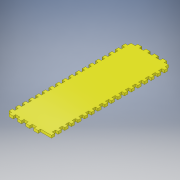
# Autodesk Inventor part: 000.203 - Боковая стенка лицевая
Saved by Autodesk Inventor 2019 (Build 230136000, 136)
## iProperties
Created: 2020-02-27
Part Number: 000.203 - Боковая стенка лицевая
Material: Типовые
Document SubType Name: Modeling
Designer: Петров Иван
Density: 1 g/cm^3
Appearance: Желтый
Author: Петров Иван
Autodesk Inventor part; units mm, degrees
ref_plane "YZ Plane" through (0, 0, 0) normal (1, 0, 0) x (0, 1, 0)
ref_plane "XZ Plane" through (0, 0, 0) normal (0, 1, 0) x (-1, 0, 0)
ref_plane "XY Plane" through (0, 0, 0) normal (0, 0, 1) x (1, 0, 0)
sketch "Эскиз1" plane through (0, 0, 0) normal (0, 1, 0) x (-1, 0, 0)
  line L0 (-22.5, 72) -> (22.5, 72)
  line L1 (22.5, 72) -> (22.5, -72)
  line L2 (22.5, -72) -> (-22.5, -72)
  line L3 (-22.5, -72) -> (-22.5, 72)
  line L4 (-22.5, 72) -> (22.5, -72) construction
  line L5 (22.5, 72) -> (-22.5, -72) construction
  point P0 (0, 0)
  point P1 (0, 0)
  dimension "d0" = 45
  dimension "d1" = 144
  constraints: 12 end point, 3 midpoint, 2 parallel, 1 horizontal, 1 perpendicular, 1 other
  measures "d0" distance of L1.end L2.end
  measures "d1" distance of L0.end L1.end
extrude "Выдавливание1" add sketch "Эскиз1" along normal blind 3
sketch "Эскиз2" plane through (0, 3, 0) normal (0, 1, 0) x (0, 0, -1)
  line L0 (-72, -22.5) -> (72, -22.5) projected
  line L1 (-72, -22.5) -> (-68, -22.5)
  line L2 (-68, -22.5) -> (-68, -25.5)
  line L3 (-68, -25.5) -> (-72, -25.5)
  line L4 (-72, -25.5) -> (-72, -22.5)
  point P0 (0, 0)
  dimension "d5" = 4
  dimension "d6" = 3
  constraints: 8 end point, 2 parallel, 1 horizontal, 1 perpendicular
  measures "d5" distance of L2.end L3.end
  measures "d6" distance of L1.end L2.end
extrude "Выдавливание2" add sketch "Эскиз2" against normal blind 3
pattern_linear "Прямоуг.массив1" count 18 spacing 8 along (0, 0, -1) of "Выдавливание2"
sketch "Эскиз3" plane through (0, 3, 0) normal (0, 1, 0) x (0, 0, -1)
  line L0 (72, 22.5) -> (-72, 22.5) projected
  line L1 (-72, 22.5) -> (-75, 22.5)
  line L2 (-75, 22.5) -> (-75, 17.5)
  line L3 (-75, 17.5) -> (-72, 17.5)
  line L4 (-72, 17.5) -> (-72, 22.5)
  line L5 (72, -22.5) -> (72, 22.5) projected
  line L6 (72, 17.5) -> (75, 17.5)
  line L7 (75, 17.5) -> (75, 12.5)
  line L8 (75, 12.5) -> (72, 12.5)
  line L9 (72, 12.5) -> (72, 17.5)
  point P0 (0, 0)
  dimension "d17" = 3
  dimension "d18" = 5
  dimension "d15" = 3
  dimension "d16" = 5
  dimension "d14" = 5
  constraints: 16 end point, 4 parallel, 2 horizontal, 2 perpendicular, 1 point on line
  measures "d17" distance of L3.end L2.end
  measures "d18" distance of L2.end L1.end
  measures "d15" distance of L7.end L8.end
  measures "d16" distance of L6.end L7.end
  measures "d14" distance between parallel lines of L0 L6
extrude "Выдавливание3" add sketch "Эскиз3" against normal blind 3
pattern_linear "Прямоуг.массив2" count 4 spacing 10 along (1, 0, 0) of "Выдавливание3"
sketch "Эскиз4" plane through (0, 3, 0) normal (0, 1, 0) x (1, 0, 0)
  line L0 (-9.4334, -33.577) -> (-9.4334, 33.2438) construction
  line L1 (-9.4334, 33.2438) -> (8.0885, 33.2438) construction
  line L2 (8.0885, 33.2438) -> (8.0885, -33.577) construction
  line L3 (8.0885, -33.577) -> (-9.4334, -33.577) construction
  point P0 (0, 0)
  constraints: 2 other
sketch "Эскиз5" plane through (0, 0, 0) normal (0, -1, 0) x (1, 0, 0)
  line L0 (-9.4334, -33.577) -> (-9.4334, 33.2438) construction
  line L1 (-9.4334, 33.2438) -> (8.0885, 33.2438) construction
  line L2 (8.0885, 33.2438) -> (8.0885, -33.577) construction
  line L3 (8.0885, -33.577) -> (-9.4334, -33.577) construction
  line L4 (8.0885, -18.72) -> (8.0885, -28.0611)
  line L5 (8.0885, -28.0611) -> (5.0082, -31.256)
  line L6 (5.0082, -31.256) -> (-6.3244, -31.256)
  line L7 (-6.3244, -31.256) -> (-9.4334, -28.0611)
  line L8 (-9.4334, -28.0611) -> (-9.4334, -18.9206)
  line L9 (-9.4334, -18.9206) -> (-8.0723, -18.9206)
  line L10 (-8.0723, -18.9206) -> (-8.0723, -27.5024)
  line L11 (-8.0723, -27.5024) -> (-5.7943, -29.852)
  line L12 (-5.7943, -29.852) -> (4.4638, -29.852)
  line L13 (4.4638, -29.852) -> (6.7418, -27.5024)
  line L14 (6.7418, -27.5024) -> (6.7418, -20.1383)
  line L15 (6.7418, -20.1383) -> (0.0224, -20.1383)
  line L16 (0.0224, -20.1383) -> (0.0224, -22.7458)
  line L17 (0.0224, -22.7458) -> (-1.353, -22.7458)
  line L18 (-1.353, -22.7458) -> (-1.353, -18.72)
  line L19 (-1.353, -18.72) -> (8.0885, -18.72)
  line L20 (8.0885, -2.0148) -> (8.0885, -14.5508)
  line L21 (8.0885, -14.5508) -> (-9.4334, -14.5508)
  line L22 (-9.4334, -14.5508) -> (-9.4334, -2.0148)
  line L23 (-9.4334, -2.0148) -> (8.0885, -2.0148)
  line L24 (6.7418, -3.4331) -> (-8.0723, -3.4331)
  line L25 (-8.0723, -3.4331) -> (-8.0723, -13.1468)
  line L26 (-8.0723, -13.1468) -> (6.7418, -13.1468)
  line L27 (6.7418, -13.1468) -> (6.7418, -3.4331)
  line L28 (4.736, 14.8767) -> (8.0885, 11.4955)
  line L29 (8.0885, 11.4955) -> (8.0885, 5.3493)
  line L30 (8.0885, 5.3493) -> (4.8649, 2.0827)
  line L31 (4.8649, 2.0827) -> (3.991, 2.9853)
  line L32 (3.991, 2.9853) -> (6.7418, 5.9224)
  line L33 (6.7418, 5.9224) -> (6.7418, 10.9081)
  line L34 (6.7418, 10.9081) -> (4.7217, 13.0858)
  line L35 (4.7217, 13.0858) -> (-6.0522, 1.9681)
  line L36 (-6.0522, 1.9681) -> (-9.4334, 5.3493)
  line L37 (-9.4334, 5.3493) -> (-9.4334, 11.4812)
  line L38 (-9.4334, 11.4812) -> (-6.1811, 14.7478)
  line L39 (-6.1811, 14.7478) -> (-5.3072, 13.8308)
  line L40 (-5.3072, 13.8308) -> (-8.0723, 10.9081)
  line L41 (-8.0723, 10.9081) -> (-8.0723, 5.9224)
  line L42 (-8.0723, 5.9224) -> (-6.0522, 3.759)
  line L43 (-6.0522, 3.759) -> (4.736, 14.8767)
  line L44 (-8.0723, 31.1951) -> (-8.0723, 25.8225)
  line L45 (-8.0723, 25.8225) -> (7.9166, 25.8225)
  line L46 (7.9166, 25.8225) -> (7.9166, 24.4184)
  line L47 (7.9166, 24.4184) -> (-8.0723, 24.4184)
  line L48 (-8.0723, 24.4184) -> (-8.0723, 19.0315)
  line L49 (-8.0723, 19.0315) -> (-9.4334, 19.0315)
  line L50 (-9.4334, 19.0315) -> (-9.4334, 31.1951)
  line L51 (-9.4334, 31.1951) -> (-8.0723, 31.1951)
  point P0 (0, 0)
  point P1 (0, 0)
  constraints: 2 other
extrude "Выдавливание4" cut sketch "Эскиз5" against normal blind 0.5
mirror "Зеркальное отражение1" about plane through (0, 0, 0) normal (1, 0, 0) of "Выдавливание2", "Прямоуг.массив1"
